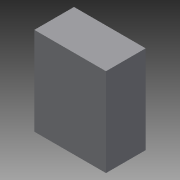
# Autodesk Inventor part: Boden
Saved by Autodesk Inventor 2014 (Build 180170000, 170)
## iProperties
Created: 2016-09-06
Part Number: Boden
Material: ABS-Kunststoff
Document SubType Name: Modeling
Designer: cem
Density: 1 g/cm^3
Appearance: Glatt - weiß
Author: cem
Autodesk Inventor part; units mm, degrees
ref_plane "YZ Plane" through (0, 0, 0) normal (1, 0, 0) x (0, 1, 0)
ref_plane "XZ Plane" through (0, 0, 0) normal (0, 1, 0) x (-1, 0, 0)
ref_plane "XY Plane" through (0, 0, 0) normal (0, 0, 1) x (1, 0, 0)
sketch "Skizze1" plane through (0, 0, 0) normal (0, 1, 0) x (-1, 0, 0)
  line L0 (49, 0) -> (-49, 0) projected
  line L1 (0, -66.5) -> (0, 66.5) projected
  line L2 (-35, 47.5) -> (35, 47.5)
  line L3 (35, 47.5) -> (35, -47.5)
  line L4 (35, -47.5) -> (-35, -47.5)
  line L5 (-35, -47.5) -> (-35, 47.5)
  point P0 (0, 0)
  dimension "d0" = 70
  dimension "d1" = 95
  constraints: 8 end point, 2 parallel, 1 horizontal, 1 perpendicular, 2 other
  measures "d0" distance between parallel lines of L3 L5
  measures "d1" distance between parallel lines of L4 L2
extrude "Extrusion1" add sketch "Skizze1" along normal blind 1
sketch "Skizze2" plane through (0, 1, 0) normal (0, 1, 0) x (1, 0, 0)
  line L0 (-35, -47.5) -> (35, -47.5) projected
  line L1 (35, -47.5) -> (35, 47.5) projected
  line L2 (35, 47.5) -> (-35, 47.5) projected
  line L3 (-35, 47.5) -> (-35, -47.5) projected
  line L4 (-33.9, 46.4) -> (33.9, 46.4)
  line L5 (33.9, 46.4) -> (33.9, -46.4)
  line L6 (33.9, -46.4) -> (-33.9, -46.4)
  line L7 (-33.9, -46.4) -> (-33.9, 46.4)
  point P0 (0, 0)
  dimension "d4" = 1.1
  constraints: 8 end point, 3 other
  measures "d4" distance between parallel lines of L1 L5
extrude "Extrusion2" add sketch "Skizze2" along normal blind 40
